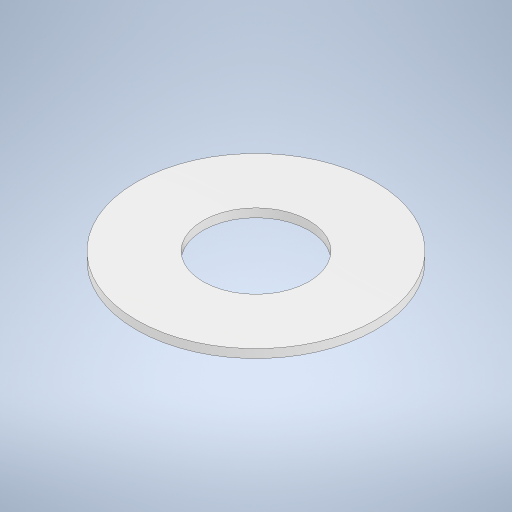
# Autodesk Inventor part: TT-0614-05
Saved by Autodesk Inventor 2024.2 (Build 282272000, 272)
## iProperties
Created: 2024-01-03
Part Number: TT-0614-05
Material: Acetal Resin, White
Document SubType Name: Modeling
Designer: Masato Kubotera
Density: 1.425 g/cm^3
Appearance: Smooth - White
Catalog Web Link: https://www.hirosugi-net.co.jp/shop/g/g31838/
Vendor: HIROSUGI
Author: Masato Kubotera
Autodesk Inventor part; units mm, degrees
ref_plane "YZ Plane" through (0, 0, 0) normal (1, 0, 0) x (0, 1, 0)
ref_plane "XZ Plane" through (0, 0, 0) normal (0, 1, 0) x (-1, 0, 0)
ref_plane "XY Plane" through (0, 0, 0) normal (0, 0, 1) x (1, 0, 0)
sketch "Sketch1" plane through (0, 0, 0) normal (0, 1, 0) x (-1, 0, 0)
  line L0 (0, 0) -> (0, 0.5)
  line L1 (-3.1, 0.5) -> (-3.1, 0)
  line L2 (-3.1, 0) -> (-7, 0)
  line L3 (-7, 0) -> (-7, 0.5)
  line L4 (-7, 0.5) -> (-3.1, 0.5)
  dimension "InsideDiameter" = 6.2
  dimension "OuterDiameter" = 14
  dimension "Thickness" = 0.5
  constraints: 10 end point, 3 vertical, 2 horizontal, 2 point on line
  measures "InsideDiameter" diameter of L1 L0
  measures "OuterDiameter" diameter of L3 L0
  measures "Thickness" distance of L2.end L3.end
revolve "Revolution1" add sketch "Sketch1" angle 360 about axis through (0, 0, 0) along (0, 0, 1)
body "Solid1"
